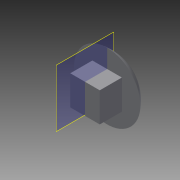
# Autodesk Inventor part: Driver Shaft Cap
Saved by Autodesk Inventor 2018 (Build 220112000, 112)
## iProperties
Created: 2018-01-21
Part Number: Driver Shaft Cap
Material: Generic
Document SubType Name: Modeling
Designer: Rus
Density: 1 g/cm^3
Appearance: Default
Author: Rus
Autodesk Inventor part; units mm, degrees
ref_plane "YZ Plane" through (0, 0, 0) normal (1, 0, 0) x (0, 1, 0)
ref_plane "XZ Plane" through (0, 0, 0) normal (0, 1, 0) x (-1, 0, 0)
ref_plane "XY Plane" through (0, 0, 0) normal (0, 0, 1) x (1, 0, 0)
sketch "Sketch1" plane through (0, 0, 0) normal (0, 0, 1) x (1, 0, 0)
  line L0 (5.6444, -5.6444) -> (-5.6444, -5.6444)
  line L1 (-5.6444, -5.6444) -> (-5.6444, 5.6444)
  line L2 (-5.6444, 5.6444) -> (5.6444, 5.6444)
  line L3 (5.6444, 5.6444) -> (5.6444, -5.6444)
  point P0 (0, 0)
  point P1 (0, 0)
  dimension "d0" = 11.2889
  constraints: 8 end point, 1 coincident, 1 horizontal, 9 other
  measures "d0" distance of L1.end L2.end
extrude "Extrusion1" add sketch "Sketch1" along normal blind 8.4667
ref_plane "Work Plane1" through (0, 5.6444, 8.4667) normal (-1, 0, 0) x (0, -1, 0)
sketch "Sketch2" plane through (0, 5.6444, 8.4667) normal (-1, 0, 0) x (0, -1, 0)
  line L0 (5.6444, -8.4667) -> (-7.0556, -8.4667)
  line L1 (0, -8.4667) -> (11.2889, -8.4667) projected
  line L2 (5.6444, -8.4667) -> (5.6444, -14.8167)
  arc A0 (-7.0556, -8.4667) -> (5.6444, -14.8167) centre (5.6444, 1.0583) ccw
  dimension "d3" = 12.7
  dimension "d4" = 6.35
  constraints: 4 end point, 2 point on circle, 1 centre point, 1 collinear, 1 line through centre, 1 vertical
  measures "d3" distance of L0.start L0.end
  measures "d4" distance of L0.start L2.end
revolve "Revolution1" add sketch "Sketch2" angle 360 about axis through (0, 0, 0) along (0, 0, -1)
body "Solid1"
